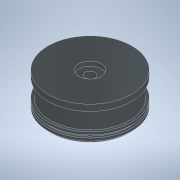
# Autodesk Inventor part: Нижняя часть поршня
Saved by Autodesk Inventor 2021 (Build 250183000, 183)
## iProperties
Created: 2020-10-24
Part Number: Нижняя часть поршня
Material: Чугун, серый
Document SubType Name: Modeling
Designer: Тимоха
Density: 7.15 g/cm^3
Appearance: Чугун серый
Mass: 59933.4 g
Surface Area: 6164.49 cm^2
Volume: 8382.29 cm^3
Author: Тимоха
Autodesk Inventor part; units mm, degrees
ref_plane "YZ Plane" through (0, 0, 0) normal (1, 0, 0) x (0, 1, 0)
ref_plane "XZ Plane" through (0, 0, 0) normal (0, 1, 0) x (-1, 0, 0)
ref_plane "XY Plane" through (0, 0, 0) normal (0, 0, 1) x (1, 0, 0)
sketch "Эскиз1" plane through (0, 0, 0) normal (0, 0, 1) x (1, 0, 0)
  line L0 (49.9998, 0) -> (189, 0)
  line L1 (137.0508, -39) -> (70.9998, -39)
  line L2 (49.9998, -20) -> (49.9998, 0)
  arc A0 (70.9998, -39) -> (54.9998, -55) centre (70.9998, -55) ccw
  arc A1 (152.99, -56.3945) -> (137.0508, -39) centre (137.0508, -55) ccw
  arc A2 (34.9998, -94) -> (24.9998, -84) centre (24.9998, -94) ccw
  line L3 (0, 0) -> (0, 25.6698)
  line L4 (149, -86) -> (152.99, -56.3945)
  line L5 (54.9998, -132) -> (54.9998, -55)
  line L6 (189, 0) -> (189, -28)
  line L7 (189, -28) -> (178, -28)
  line L8 (178, -28) -> (178, -108)
  line L9 (178, -108) -> (189, -108)
  line L10 (189, -108) -> (189, -120)
  line L11 (189, -120) -> (178, -120)
  line L12 (178, -120) -> (178, -132)
  line L13 (178, -132) -> (189, -132)
  line L14 (189, -132) -> (189, -144)
  line L15 (189, -144) -> (178, -144)
  line L16 (178, -144) -> (178, -156)
  line L17 (178, -156) -> (158, -156)
  line L18 (158, -156) -> (158, -148)
  line L19 (158, -148) -> (149, -148)
  line L20 (149, -86) -> (149, -148)
  line L21 (24.9998, -84) -> (22.4998, -84)
  line L22 (22.4998, -84) -> (22.4998, -20)
  line L23 (22.4998, -20) -> (49.9998, -20)
  line L24 (34.9998, -94) -> (34.9998, -156)
  line L25 (34.9998, -156) -> (39.9998, -156)
  line L26 (39.9998, -156) -> (39.9998, -148)
  line L27 (39.9998, -148) -> (54.9998, -148)
  line L28 (54.9998, -148) -> (54.9998, -132)
  point P0 (154.5118, -39)
  point P1 (54.9998, -39)
  point P2 (34.9998, -84)
  dimension "d0" = 189
  dimension "d5" = 99.512
  dimension "d9" = 16
  dimension "d10" = 16
  dimension "d11" = 10
  dimension "d29" = 20
  dimension "d30" = 28
  dimension "d31" = 11
  dimension "d32" = 80
  dimension "d34" = 12
  dimension "d35" = 11
  dimension "d36" = 12
  dimension "d37" = 11
  dimension "d38" = 12
  dimension "d39" = 11
  dimension "d40" = 12
  dimension "d41" = 20
  dimension "d42" = 8
  dimension "d43" = 2.5
  dimension "d44" = 64
  constraints: 58 end point, 10 perpendicular, 6 point on circle, 6 vertical, 5 horizontal, 4 point on line, 3 centre point, 2 tangent, 1 collinear
  measures "d0" distance of L3.start L0.end
  measures "d5" distance of point (154.512, -39) point (55, -39)
  measures "d9" radius of A0
  measures "d10" radius of A1
  measures "d11" radius of A2
  measures "d29" distance of L2.start L2.end
  measures "d30" distance of L0.end L6.end
  measures "d31" distance of L6.end L7.end
  measures "d32" distance of L7.end L8.end
  measures "d34" distance of L9.end L10.end
  measures "d35" distance of L10.end L11.end
  measures "d36" distance of L11.end L12.end
  measures "d37" distance of L12.end L13.end
  measures "d38" distance of L13.end L14.end
  measures "d39" distance of L14.end L15.end
  measures "d40" distance of L15.end L16.end
  measures "d41" distance of L16.end L17.end
  measures "d42" distance of L17.end L18.end
  measures "d43" distance of L21.start L21.end
  measures "d44" distance of L21.end L22.end
revolve "Вращение1" add sketch "Эскиз1" angle 360 about axis through (0, 0, 0) along (0, 1, 0)
